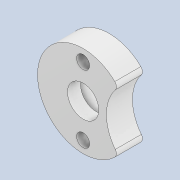
# Autodesk Inventor part: Suport_Rulment
Saved by Autodesk Inventor 2020 (Build 240168000, 168)
## iProperties
Created: 2021-02-03
Part Number: Suport_Rulment
Material: ABS Plastic
Document SubType Name: Modeling
Designer: Iulian Bors
Density: 1.06 g/cm^3
Appearance: Smooth - White
Mass: 6.87038 g
Surface Area: 33.129 cm^2
Volume: 6.48149 cm^3
Description: Suport_Rulment
Author: Iulian Bors
Subject: 005
Autodesk Inventor part; units mm, degrees
ref_plane "YZ Plane" through (0, 0, 0) normal (1, 0, 0) x (0, 1, 0)
ref_plane "XZ Plane" through (0, 0, 0) normal (0, 1, 0) x (-1, 0, 0)
ref_plane "XY Plane" through (0, 0, 0) normal (0, 0, 1) x (1, 0, 0)
sketch "Sketch1" plane through (0, 0, 0) normal (0, 0, 1) x (1, 0, 0)
  circle A0 centre (0, 0) radius 6
  circle A1 centre (0, 0) radius 17.5
  dimension "d0" = 12
  dimension "d1" = 35
  constraints: 2 centre point, 2 coincident
  measures "d0" diameter of A0
  measures "d1" diameter of A1
extrude "Extrusion1" add sketch "Sketch1" along normal blind 10
sketch "Sketch4" plane through (0, 0, 0) normal (0, 0, -1) x (-1, 0, 0)
  circle A0 centre (0, 0) radius 13 construction
  point P0 (0, -13)
  point P1 (0, 13)
  dimension "d7" = 26
  constraints: 2 point on circle, 2 vertical alignment, 1 centre point, 1 coincident
  measures "d7" diameter of A0
hole "Hole1" at (0, -13, 0) at (0, 13, 0) direction (0, 0, 1) diameter 5 end through all
sketch "Sketch5" plane through (0, 0, 0) normal (0, 0, -1) x (-1, 0, 0)
  circle A0 centre (0, 0) radius 8.15
  dimension "d15" = 16.3
  constraints: 1 centre point, 1 coincident
  measures "d15" diameter of A0
extrude "Extrusion3" cut sketch "Sketch5" against normal blind 5
sketch "Sketch6" plane through (0, 0, 10) normal (0, 0, 1) x (1, 0, 0)
  arc A0 (25.0591, 16.1) -> (25.0591, -16.1) centre (25.0591, 0) ccw projected
  arc A1 (25.0591, 17.1) -> (25.0591, -17.1) centre (25.0591, 0) ccw
  circle A2 centre (0, 0) radius 17.5 projected
  point P0 (12.8057, 11.9274)
  point P1 (12.8057, -11.9274)
  point P2 (13.4681, 11.174)
  point P3 (13.4681, -11.174)
  dimension "d22" = 1
  constraints: 2 point on circle, 1 centre point
  measures "d22" radial gap between concentric circles of A0 A1
extrude "Extrusion4" cut sketch "Sketch6" against normal through all contours A2 A0
fillet "Fillet1" radius 2 2 edges at (13.4681, -11.174, 5) (13.4681, 11.174, 5)
body "Solid1"
